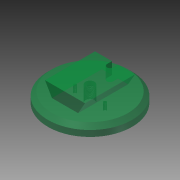
# Autodesk Inventor part: 13_1087_061
Saved by Autodesk Inventor 2014 SP1 (Build 180222100, 222)
## iProperties
Created: 2013-09-18
Part Number: 13_1087_061
Material: Allgemein
Document SubType Name: Modeling
Designer: vogel
Density: 1 g/cm^3
Appearance: Klar - grün 1
Author: vogel
Autodesk Inventor part; units mm, degrees
ref_plane "YZ Plane" through (0, 0, 0) normal (1, 0, 0) x (0, 1, 0)
ref_plane "XY Plane" through (0, 0, 0) normal (0, 0, 1) x (1, 0, 0)
sketch "Skizze1" plane through (0, 0, 0) normal (0, 0, 1) x (1, 0, 0)
  line L0 (-29.4, 0) -> (29.4, 0) projected
  line L1 (0, -29.4) -> (0, 29.4) projected
  circle A0 centre (0, 0) radius 21
  circle A1 centre (0, 0) radius 19.5
  dimension "d0" = 42
  dimension "d1" = 39
  constraints: 2 centre point, 2 coincident
  measures "d0" diameter of A0
  measures "d1" diameter of A1
extrude "Extrusion1" add sketch "Skizze1" along normal blind 40 contours A1 L1 A0 L0 | L0 A0 L1 A1 | A1 L0 A0 L1 | L1 A0 L0 A1
sketch "Skizze2" plane through (0, 0, 40) normal (0, 0, 1) x (1, 0, 0)
  circle A0 centre (0, 0) radius 19.5 projected
extrude "Extrusion2" add sketch "Skizze2" against normal blind 1
sketch "Skizze3" plane through (0, 0, 40) normal (0, 0, 1) x (1, 0, 0)
  circle A0 centre (0, 0) radius 21 projected
extrude "Extrusion3" add sketch "Skizze3" along normal blind 4
sketch "Skizze4" plane through (0, 0, 0) normal (0, 1, 0) x (-1, 0, 0)
  line L0 (21, 44) -> (-21, 44) projected
  line L1 (10, 50) -> (-10, 50)
  line L2 (0, -9.2) -> (0, 55.2) projected
  line L3 (29.4, 0) -> (-29.4, 0) projected
  line L4 (-10, 50) -> (-6.5359, 44)
  line L5 (10, 50) -> (6.5359, 44)
  line L6 (-6.5359, 44) -> (6.5359, 44)
  point P0 (0, 0)
  dimension "d8" = 20
  dimension "d9" = 6
  dimension "d10" = 60
  constraints: 8 end point, 2 parallel, 2 point on line, 1 other
  measures "d8" distance of L1.start L1.end
  measures "d9" vertical distance of L1.end L4.end
  measures "d10" angle of L1 L4
extrude "Extrusion4" add sketch "Skizze4" along normal mid plane 25
ref_plane "Arbeitsebene1" through (0, 21, 0) normal (0, 1, 0) x (-1, 0, 0)
sketch "Skizze5" plane through (0, 21, 0) normal (0, 1, 0) x (-1, 0, 0)
  line L0 (29.4, 0) -> (-29.4, 0) projected
  line L1 (0, -10) -> (0, 60) projected
  point P0 (0, 0)
  point P1 (0, 2)
  dimension "d16" = 2
  constraints: 1 point on line
  measures "d16" distance from line of point (0, 2) L0
hole "Bohrung1" at (0, 21, 2) direction (0, -1, 0) diameter 2.4 end through all
pattern_circular "Runde Anordnung1" count 4 over 360 about axis through (0, 0, 0) along (0, 0, 1) of "Bohrung1"
sketch "Skizze6" plane through (-10, 12.5, 50) normal (0, 0, 1) x (1, 0, 0)
  line L0 (0, 0) -> (20, 0) projected
  line L1 (-19.4018, -12.5) -> (39.4018, -12.5) projected
  line L2 (10, -41.9018) -> (10, 16.9018) projected
  circle A0 centre (10, -2.5) radius 1.5
  line L3 (8.5, -2.5) -> (8.5, 0)
  line L4 (11.5, -2.5) -> (11.5, 0)
  line L5 (11.5, 0) -> (8.5, 0)
  point P0 (10, -12.5)
  dimension "d27" = 10
  dimension "d28" = 3
  constraints: 6 end point, 3 point on line, 2 perpendicular, 2 point on circle, 2 tangent, 1 centre point, 1 collinear
  measures "d27" distance from line of A0.centre L1
  measures "d28" diameter of A0
extrude "Extrusion5" cut sketch "Skizze6" against normal up to surface (6 mm away)
chamfer "Fase2" distance 2 angle 45 1 edges at (-21, 0, 44)
sketch "Skizze8" plane through (0, 0, 0) normal (0, 0, -1) x (-1, 0, 0)
  circle A0 centre (0, 0) radius 19.5 projected
  circle A1 centre (0, 0) radius 21 projected
extrude "Extrusion6" cut sketch "Skizze8" against normal up to surface (39 mm away)
sketch "Skizze9" plane through (0, 0, 39) normal (0, 0, -1) x (-1, 0, 0)
  circle A0 centre (0, 0) radius 21 projected
  constraints: 1 coincident
hole "Bohrung2" at (0, 0, 39) direction (0, 0, 1) diameter 4.459 depth 8 tip angle 118 thread size "M5x0.5" class "6H" standard "ISO Metric profile"
sketch "Skizze11" plane through (0, 0, 39) normal (0, 0, -1) x (-1, 0, 0)
  circle A0 centre (0, 0) radius 21 projected
  circle A1 centre (0, 0) radius 7.5
  line L0 (29.4, 0) -> (-29.4, 0) projected
  line L1 (0, -29.4) -> (0, 29.4) projected
  point P0 (-7.5, 0)
  point P1 (7.5, 0)
  dimension "d44" = 15
  constraints: 2 point on circle, 2 point on line, 1 centre point, 1 coincident
  measures "d44" diameter of A1
hole "Bohrung3" at (7.5, 0, 39) at (-7.5, 0, 39) direction (0, 0, 1) diameter 1.567 depth 4 tip angle 118 thread size "M2x0.4" class "6H" standard "ISO Metric profile"
